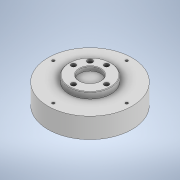
# Autodesk Inventor part: マニピュレータ手首ISO9409
Saved by Autodesk Inventor 2021 (Build 250183000, 183)
## iProperties
Created: 2021-09-24
Part Number: マニピュレータ手首ISO9409
Material: 一般
Document SubType Name: Modeling
Designer: tomat
Density: 1 g/cm^3
Appearance: 既定
Author: tomat
Autodesk Inventor part; units mm, degrees
ref_plane "YZ Plane" through (0, 0, 0) normal (1, 0, 0) x (0, 1, 0)
ref_plane "XZ Plane" through (0, 0, 0) normal (0, 1, 0) x (-1, 0, 0)
ref_plane "XY Plane" through (0, 0, 0) normal (0, 0, 1) x (1, 0, 0)
sketch "スケッチ1" plane through (0, 0, 0) normal (0, 0, 1) x (1, 0, 0)
  line L0 (0, 0) -> (40, 0)
  line L1 (40, 0) -> (40, 19.3)
  line L2 (40, 19.3) -> (20, 19.3)
  line L3 (20, 19.3) -> (20, 25.3)
  line L4 (20, 25.3) -> (0, 25.3)
  line L5 (0, 25.3) -> (0, 0)
  line L6 (20, 24.8) -> (19.5, 25.3)
  line L7 (10, 25.3) -> (10, 21.3)
  line L8 (10, 21.3) -> (0, 21.3)
  line L9 (10.5, 25.3) -> (10, 24.8)
  dimension "d0" = 40
  dimension "d1" = 19.3
  dimension "d2" = 20
  dimension "d3" = 6
  dimension "d4" = 135
  dimension "d5" = 0.5
  dimension "d6" = 4
  dimension "d7" = 0.5
  dimension "d8" = 45
  constraints: 20 end point, 6 perpendicular, 5 point on line, 1 horizontal, 1 midpoint, 1 vertical
  measures "d0" distance of L0.start L0.end
  measures "d1" distance of L0.end L1.end
  measures "d2" distance of L1.end L2.end
  measures "d3" distance of L2.end L3.end
  measures "d4" angle of L3 L6
  measures "d5" distance of L3.end L6.start
  measures "d6" distance of L7.start L7.end
  measures "d7" distance of L7.start L9.start
  measures "d8" angle of L4 L9
revolve "回転1" add sketch "スケッチ1" angle 360 about axis through (0, 25.3, 0) along (0, -1, 0) contours L5 L8 L7 L9 L4 L6 L3 L2 L1 L0
sketch "スケッチ2" plane through (0, 19.3, 0) normal (0, 1, 0) x (1, 0, 0)
  point P0 (0, 0)
  point P1 (0, -35)
  point P2 (0, 0)
  point P3 (35, 0)
  point P4 (0, 35)
  point P5 (-35, 0)
  dimension "d12" = 360
  constraints: 1 coincident, 5 other
hole "穴1" at (0, 19.3, 35) at (0, 19.3, 0) at (35, 19.3, 0) at (0, 19.3, -35) at (-35, 19.3, 0) direction (0, -1, 0) diameter 2.459 depth 6 tip angle 118 thread size "M3x0.5" class "6H" standard "ISO Metric profile"
sketch "スケッチ3" plane through (0, 25.3, 0) normal (0, 1, 0) x (1, 0, 0)
  point P0 (0, 0)
  point P1 (0, 15.75)
  point P2 (-15.75, 0)
  point P3 (0, -15.75)
  point P4 (15.75, 0)
  dimension "d21" = 15.75
  dimension "d24" = 360
  constraints: 5 other
  measures "d21" distance of point (0, 0) point (0, 15.75)
hole "穴2" at (0, 25.3, -15.75) at (-15.75, 25.3, 0) at (0, 25.3, 15.75) at (15.75, 25.3, 0) direction (0, -1, 0) diameter 4.4587 depth 8 tip angle 118 thread size "M5x0.5" class "6H" standard "ISO Metric profile"
sketch "スケッチ4" plane through (0, 25.3, 0) normal (0, 1, 0) x (1, 0, 0)
  circle A0 centre (0, 0) radius 1.2295 projected
  circle A1 centre (0, 0) radius 15.75 construction
  line L0 (-11.1369, 11.1369) -> (0, 0) construction
  line L1 (0, 0) -> (-15.75, 0) construction
  dimension "d33" = 31.5
  dimension "d34" = 45
  constraints: 4 end point, 2 point on circle, 1 centre point, 1 coincident, 1 horizontal
  measures "d33" diameter of A1
  measures "d34" angle of L1 L0
hole "穴3" at (-11.1369, 25.3, -11.1369) direction (0, -1, 0) diameter 5 depth 8 tip angle 118
